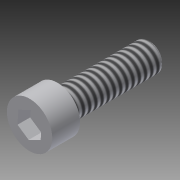
# Autodesk Inventor part: 4_40_hex_cap_screw
Saved by Autodesk Inventor 2014 (Build 180170000, 170)
## iProperties
Created: 2014-03-24
Part Number: 4_40_hex_cap_screw
Material: Generic
Document SubType Name: Modeling
Designer: stephenholtz
Density: 1 g/cm^3
Appearance: Default
Author: stephenholtz
Autodesk Inventor part; units mm, degrees
ref_plane "YZ Plane" through (0, 0, 0) normal (1, 0, 0) x (0, 1, 0)
ref_plane "XZ Plane" through (0, 0, 0) normal (0, 1, 0) x (-1, 0, 0)
ref_plane "XY Plane" through (0, 0, 0) normal (0, 0, 1) x (1, 0, 0)
sketch "Sketch1" plane through (0, 0, 0) normal (0, 0, 1) x (1, 0, 0)
  circle A0 centre (0, 0) radius 2.3241
  dimension "max_head_dia" = 4.6482
  constraints: 1 centre point, 1 coincident
  measures "max_head_dia" diameter of A0
extrude "Extrusion1" add sketch "Sketch1" along normal blind 2.8448
sketch "Sketch2" plane through (0, 0, 0) normal (0, 0, -1) x (-1, 0, 0)
  circle A0 centre (0, 0) radius 2.3241 projected
  circle A1 centre (0, 0) radius 1.4224
  dimension "max_body_dia" = 2.8448
  constraints: 1 centre point, 1 coincident
  measures "max_body_dia" diameter of A1
extrude "Extrusion2" add sketch "Sketch2" along normal blind 9.525 contours A1
sketch "Sketch3" plane through (0, 0, 2.8448) normal (0, 0, 1) x (1, 0, 0)
  circle A0 centre (0, 0) radius 2.3241 projected
  line L0 (-1.1397, 0.7689) -> (0.096, 1.3715)
  line L1 (0.096, 1.3715) -> (1.2357, 0.6026)
  line L2 (1.2357, 0.6026) -> (1.1397, -0.7689)
  line L3 (1.1397, -0.7689) -> (-0.096, -1.3715)
  line L4 (-0.096, -1.3715) -> (-1.2357, -0.6026)
  line L5 (-1.2357, -0.6026) -> (-1.1397, 0.7689)
  dimension "hex_socket_size" = 2.3813
  constraints: 12 end point, 1 coincident, 13 other
  measures "hex_socket_size" distance between parallel lines of L3 L0
extrude "Extrusion3" cut sketch "Sketch3" against normal blind 1.2954 contours L0 L1 L2 L3 L4 L5
thread "Thread1" size "4-40 UNC" class "2A" standard "ANSI Unified Screw Threads" full length
chamfer "Chamfer1" distance 0.254 angle 45 1 edges at (1.4224, 0, -9.525)
body "Solid1"
